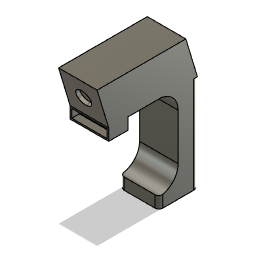
thermal + barcode device v1 (Autodesk Fusion 360 design; units mm, degrees)
Autodesk Fusion 360 part; units mm, degrees
sketch "Sketch1" plane through (0, 0, 0) normal (0, 1, 0) x (1, 0, 0)
  line L0 (-20, 25) -> (20, 25)
  line L1 (25, 20) -> (25, -20)
  line L2 (20, -25) -> (-20, -25)
  line L3 (-25, -20) -> (-25, 20)
  arc A0 (-20, 25) -> (-25, 20) centre (-20, 20) ccw
  arc A1 (25, 20) -> (20, 25) centre (20, 20) ccw
  arc A2 (-25, -20) -> (-20, -25) centre (-20, -20) ccw
  arc A3 (20, -25) -> (25, -20) centre (20, -20) ccw
  dimension "d1" = 5
  dimension "d2" = 5
  dimension "d3" = 5
  dimension "d4" = 5
  constraint horizontal L0
  constraint vertical L1
  constraint horizontal L2
  constraint vertical L3
  constraint tangent L3 A0
  constraint tangent L0 A0
  constraint tangent L0 A1
  constraint tangent L1 A1
  constraint tangent L2 A2
  constraint tangent L3 A2
  constraint tangent L2 A3
  constraint tangent L1 A3
  measures "d1" radius of A0
  measures "d2" radius of A1
  measures "d3" radius of A2
  measures "d4" radius of A3
extrude "Extrude1" add sketch "Sketch1" along normal blind 15
sketch "Sketch2" plane through (-25, 0, 0) normal (-1, 0, 0) x (0, 0, 1)
  line L0 (-20, 0) -> (20, 0)
  line L1 (20, 0) -> (20, 15)
  line L2 (20, 15) -> (-20, 15)
  line L3 (-20, 15) -> (-20, 0)
  line L4 (-25, 15) -> (-25, 125)
  arc A0 (0, 40) -> (25, 15) centre (25, 40) ccw
  arc A1 (25, 125) -> (0, 100) centre (25, 100) ccw
  line L5 (0, 40) -> (0, 100)
  line L6 (25, 125) -> (-25, 125)
  line L7 (25, 15) -> (-25, 15)
  constraint perpendicular L2 L4
  constraint tangent L2 A0
  constraint tangent A1 L5
  constraint tangent A1 L6
  constraint tangent A0 L7
extrude "Extrude2" add sketch "Sketch2" against normal blind 50 contours L2 L4 A0 A1 L5 L6 L7
extrude "Extrude3" cut 1 faces at (-24.0177, 15, 24.0177) along direction (0, 1, 0) blind 5
extrude "Extrude4" cut 3 faces at (24.0177, 15, 24.0177) (24.0177, 15, -24.0177) (-24.0177, 15, -24.0177) along direction (0, 1, 0) blind 160
box "BoxPrimitive1" add length 50 width 50 height 50 placed x (0, 0, 1) y (1, 0, 0) z (0, 1, 0) at (-25, 125, -25)
sketch "Sketch4" plane through (-25, 0, 0) normal (-1, 0, 0) x (0, 0, 1)
  line L0 (-20, 125) -> (-20, 0)
  line L1 (-20, 0) -> (20, 0)
  line L2 (20, 0) -> (20, 15.5051)
  arc A0 (0, 40) -> (20, 15.5051) centre (25, 40) ccw
  line L3 (0, 40) -> (0, 100)
  arc A1 (25, 125) -> (0, 100) centre (25, 100) ccw
  line L4 (25, 125) -> (25, 175)
  line L5 (25, 175) -> (-25, 175)
  line L6 (-25, 175) -> (-25, 125)
  line L7 (-25, 125) -> (-20, 125)
  line L8 (-25, 125) -> (-10, 175)
  constraint coincident L6.end L7.start
  constraint coincident L5 L8.end
extrude "Extrude5" cut sketch "Sketch4" against normal blind 60 contours L5 L6 L8
sketch "Sketch5" plane through (0, 17.2018, -57.3394) normal (0, 0.287348, -0.957826) x (-1, 0, 0)
  line L0 (-25, 164.7461) -> (-25, 112.5446)
  line L1 (-25, 112.5446) -> (-20, 112.5446)
  line L2 (-20, 112.5446) -> (20, 112.5446)
  line L3 (20, 112.5446) -> (25, 112.5446)
  line L4 (25, 112.5446) -> (25, 164.7461)
  line L5 (25, 164.7461) -> (-25, 164.7461)
  line L6 (-25, 164.7461) -> (25, 164.7461)
  line L7 (25, 164.7461) -> (25, 112.5446)
  line L8 (25, 112.5446) -> (-25, 112.5446)
  line L9 (-25, 112.5446) -> (-25, 164.7461)
  line L10 (23, 114.5446) -> (-23, 114.5446)
  line L11 (-23, 114.5446) -> (-23, 162.7461)
  line L12 (-23, 162.7461) -> (23, 162.7461)
  line L13 (23, 162.7461) -> (23, 114.5446)
  dimension "d20" = 2
  constraint horizontal L6
  constraint vertical L7
  constraint horizontal L8
  constraint vertical L9
  constraint coincident L3.end L4.start
  constraint coincident L0.start L5.end
extrude "Extrude6" cut sketch "Sketch5" against normal blind 5 contours L10 L11 L12 L13
extrude "Extrude7" add 1 faces at (6.6667, 158.3333, 25) along direction (0, 0, 1) blind 80
sketch "Sketch6" plane through (-25, 0, 0) normal (-1, 0, 0) x (0, 0, 1)
  line L0 (-10, 175) -> (-25, 125)
  line L1 (-25, 125) -> (-20, 125)
  line L2 (-20, 125) -> (-20, 0)
  line L3 (-20, 0) -> (20, 0)
  line L4 (20, 0) -> (20, 15.5051)
  arc A0 (0, 40) -> (20, 15.5051) centre (25, 40) ccw
  line L5 (0, 40) -> (0, 100)
  arc A1 (25, 125) -> (0, 100) centre (25, 100) ccw
  line L6 (25, 125) -> (105, 125)
  line L7 (105, 125) -> (105, 175)
  line L8 (105, 175) -> (-10, 175)
  line L9 (105, 175) -> (90, 125)
  constraint coincident L7.end L8.start
  constraint coincident L6 L9.end
extrude "Extrude8" cut sketch "Sketch6" against normal blind 85 contours L6 L7 L9
sketch "Sketch7" plane through (0, -14.4495, 48.1651) normal (0, -0.287348, 0.957826) x (1, 0, 0)
  line L0 (25, 145.5896) -> (25, 197.7911)
  line L1 (25, 197.7911) -> (-25, 197.7911)
  line L2 (-25, 197.7911) -> (-25, 145.5896)
  line L3 (-25, 145.5896) -> (25, 145.5896)
  line L4 (-25, 197.7911) -> (25, 197.7911)
  line L5 (25, 197.7911) -> (25, 145.5896)
  line L6 (25, 145.5896) -> (-25, 145.5896)
  line L7 (-25, 145.5896) -> (-25, 197.7911)
  circle A0 centre (0, 171.6904) radius 10
  dimension "d27" = 20
  constraint horizontal L4
  constraint vertical L5
  constraint horizontal L6
  constraint vertical L7
  constraint coincident L0.start L3.end
  constraint coincident L1.end L2.start
  measures "d27" diameter of A0
extrude "Extrude9" cut sketch "Sketch7" against normal blind 5 contours A0
sketch "Sketch8" plane through (0, 125, 0) normal (0, -1, 0) x (1, 0, 0)
  line L0 (25, 90) -> (-25, 90)
  line L1 (-25, 90) -> (-25, 25)
  line L2 (-25, 25) -> (20, 25)
  arc A0 (25, 20) -> (20, 25) centre (20, 20) ccw
  line L3 (25, 20) -> (25, 90)
  line L4 (-25, 90) -> (25, 90)
  line L5 (25, 90) -> (25, 65)
  line L6 (25, 65) -> (-25, 65)
  line L7 (-25, 65) -> (-25, 90)
  constraint horizontal L4
  constraint vertical L5
  constraint horizontal L6
  constraint vertical L7
  constraint coincident L3 L5.end
  constraint coincident L0.end L1.start
extrude "Extrude10" add sketch "Sketch8" along normal blind 15 contours L0 L1 L3 L4 L5 L6 L7
sketch "Sketch9" plane through (0, 0, 90) normal (0, 0, 1) x (1, 0, 0)
  line L0 (25, 125) -> (-25, 125)
  line L1 (-25, 125) -> (-25, 110)
  line L2 (-25, 110) -> (25, 110)
  line L3 (25, 110) -> (25, 125)
  line L4 (-25, 125) -> (25, 125)
  line L5 (25, 125) -> (25, 110)
  line L6 (25, 110) -> (-25, 110)
  line L7 (-25, 110) -> (-25, 125)
  line L8 (23, 112) -> (-23, 112)
  line L9 (-23, 112) -> (-23, 123)
  line L10 (-23, 123) -> (23, 123)
  line L11 (23, 123) -> (23, 112)
  dimension "d32" = 2
  constraint horizontal L4
  constraint vertical L5
  constraint horizontal L6
  constraint vertical L7
  constraint coincident L2.end L3.start
  constraint coincident L0.end L1.start
extrude "Extrude11" cut sketch "Sketch9" against normal blind 10 contours L8 L9 L10 L11
